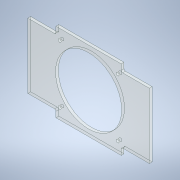
# Autodesk Inventor part: Schutzglas_Lüfter
Saved by Autodesk Inventor 2022 (Build 260153000, 153)
## iProperties
Created: 2021-04-28
Part Number: Schutzglas_Lüfter
Material: Glas
Document SubType Name: Modeling
Designer: Sebastian Seewald
Density: 2.18 g/cm^3
Appearance: Klar
Author: Sebastian Seewald
Autodesk Inventor part; units mm, degrees
ref_plane "YZ Plane" through (0, 0, 0) normal (1, 0, 0) x (0, 1, 0)
ref_plane "XZ Plane" through (0, 0, 0) normal (0, 1, 0) x (-1, 0, 0)
ref_plane "XY Plane" through (0, 0, 0) normal (0, 0, 1) x (1, 0, 0)
sketch "Skizze1" plane through (0, 0, 0) normal (0, 0, 1) x (1, 0, 0)
  line L0 (-86.35, 56.35) -> (86.35, 56.35)
  line L1 (86.35, 56.35) -> (86.35, -56.35)
  line L2 (86.35, -56.35) -> (-86.35, -56.35)
  line L3 (-86.35, -56.35) -> (-86.35, 56.35)
  line L4 (-86.35, 56.35) -> (86.35, -56.35) construction
  line L5 (86.35, 56.35) -> (-86.35, -56.35) construction
  point P0 (0, 0)
  dimension "d0" = 172.7
  dimension "d1" = 112.7
  constraints: 12 end point, 2 midpoint, 2 parallel, 1 horizontal, 1 perpendicular
  measures "d0" distance between parallel lines of L3 L1
  measures "d1" distance of L2.end L0.start
extrude "Extrusion1" add sketch "Skizze1" along normal blind 4
sketch "Skizze2" plane through (0, 0, 4) normal (0, 0, 1) x (1, 0, 0)
  circle A0 centre (0, 0) radius 47
  dimension "d4" = 94
  constraints: 1 centre point, 1 coincident
  measures "d4" diameter of A0
extrude "Extrusion2" cut sketch "Skizze2" against normal blind 4
sketch "Skizze3" plane through (0, 0, 4) normal (0, 0, 1) x (1, 0, 0)
  circle A0 centre (-41.25, 41.25) radius 2.2
  circle A1 centre (41.25, 41.25) radius 2.2
  circle A2 centre (41.25, -41.25) radius 2.2
  circle A3 centre (-41.25, -41.25) radius 2.2
  point P0 (0, 0)
  dimension "d7" = 82.5
  dimension "d8" = 82.5
  dimension "d9" = 82.5
  dimension "d10" = 82.5
  dimension "d11" = 41.25
  dimension "d12" = 41.25
  dimension "d13" = 41.25
  dimension "d14" = 41.25
  dimension "d15" = 4.4
  dimension "d16" = 4.4
  dimension "d17" = 4.4
  dimension "d18" = 4.4
  constraints: 4 centre point
  measures "d7" distance of A1.centre A0.centre
  measures "d8" distance of A3.centre A2.centre
  measures "d9" distance of A3.centre A0.centre
  measures "d10" distance of A1.centre A2.centre
  measures "d11" horizontal distance of point (0, 0) A0.centre
  measures "d12" horizontal distance of point (0, 0) A1.centre
  measures "d13" horizontal distance of point (0, 0) A3.centre
  measures "d14" horizontal distance of point (0, 0) A2.centre
  measures "d15" diameter of A0
  measures "d16" diameter of A1
  measures "d17" diameter of A2
  measures "d18" diameter of A3
extrude "Extrusion3" cut sketch "Skizze3" against normal blind 4
sketch "Skizze4" plane through (0, 0, 4) normal (0, 0, 1) x (1, 0, 0)
  line L0 (-86.35, 56.35) -> (-46.35, 56.35)
  line L1 (-46.35, 56.35) -> (-46.35, 46.35)
  line L2 (-46.35, 46.35) -> (-86.35, 46.35)
  line L3 (-86.35, 46.35) -> (-86.35, 56.35)
  line L4 (86.35, -56.35) -> (86.35, 56.35) projected
  line L5 (86.35, 56.35) -> (46.35, 56.35)
  line L6 (46.35, 56.35) -> (46.35, 46.35)
  line L7 (46.35, 46.35) -> (86.35, 46.35)
  line L8 (86.35, 46.35) -> (86.35, 56.35)
  line L9 (86.35, -56.35) -> (46.35, -56.35)
  line L10 (46.35, -56.35) -> (46.35, -46.35)
  line L11 (46.35, -46.35) -> (86.35, -46.35)
  line L12 (86.35, -46.35) -> (86.35, -56.35)
  line L13 (-86.35, -56.35) -> (86.35, -56.35) projected
  line L14 (-86.35, -56.35) -> (-46.35, -56.35)
  line L15 (-46.35, -56.35) -> (-46.35, -46.35)
  line L16 (-46.35, -46.35) -> (-86.35, -46.35)
  line L17 (-86.35, -46.35) -> (-86.35, -56.35)
  line L18 (-86.35, 56.35) -> (-86.35, -56.35) projected
  point P0 (86.35, -46.35)
  point P1 (86.35, 46.35)
  dimension "d31" = 40
  dimension "d32" = 40
  dimension "d33" = 10
  dimension "d34" = 10
  constraints: 32 end point, 8 parallel, 4 horizontal, 4 perpendicular, 4 point on line
  measures "d31" distance between parallel lines of L18 L1
  measures "d32" distance between parallel lines of L4 L6
  measures "d33" distance between parallel lines of L13 L11
  measures "d34" distance between parallel lines of L5 L7
extrude "Extrusion4" cut sketch "Skizze4" against normal blind 10
fillet "Rundung1" radius 2 4 edges at (-46.35, 46.35, 2) (46.35, 46.35, 2) (46.35, -46.35, 2) (-46.35, -46.35, 2)
